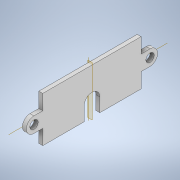
# Autodesk Inventor part: pokrywa_baza
Saved by Autodesk Inventor 2021 (Build 250183000, 183)
## iProperties
Created: 2025-11-29
Part Number: pokrywa_baza
Material: Generic
Document SubType Name: Modeling
Designer: huber
Density: 1 g/cm^3
Appearance: Default
Author: huber
Autodesk Inventor part; units mm, degrees
ref_plane "YZ Plane" through (0, 0, 0) normal (1, 0, 0) x (0, 1, 0)
ref_plane "XZ Plane" through (0, 0, 0) normal (0, 1, 0) x (-1, 0, 0)
sketch "Sketch1" plane through (0, 0, 0) normal (1, 0, 0) x (0, 1, 0)
  line L0 (11.5, 25) -> (-11.5, 25)
  line L1 (-11.5, 25) -> (-11.5, -25)
  line L2 (-11.5, -25) -> (11.5, -25)
  line L3 (11.5, -25) -> (11.5, 25)
  line L4 (11.5, 25) -> (-11.5, -25) construction
  line L5 (-11.5, 25) -> (11.5, -25) construction
  circle A0 centre (0, -29.5) radius 3.875
  line L6 (3.875, -29.5) -> (3.875, -25)
  line L7 (-3.875, -29.5) -> (-3.875, -25)
  line L8 (0, -45.05) -> (0, 36.675) projected
  circle A1 centre (0, -29.5) radius 2.1
  line L9 (-16.1, 0) -> (16.1, 0) projected
  circle A2 centre (-4.5, 0) radius 4
  line L10 (-4.5, 4) -> (-11.5, 4)
  line L11 (-4.5, -4) -> (-11.5, -4)
  point P0 (0, 0)
  point P1 (-11.5, 1.75)
  point P2 (-11.5, -4.25)
  point P3 (4, 25)
  point P4 (-4, 25)
  dimension "d0" = 50
  dimension "d1" = 23
  dimension "d4" = 7.75
  dimension "d5" = 4.5
  dimension "d6" = 4.2
  dimension "d11" = 8
  dimension "d12" = 7
  constraints: 20 end point, 10 point on line, 5 perpendicular, 4 point on circle, 4 tangent, 3 centre point, 2 midpoint, 2 parallel, 1 coincident, 1 horizontal
  measures "d0" distance of L0.end L1.end
  measures "d1" distance of L1.end L2.end
  measures "d4" diameter of A0
  measures "d5" distance from line of L2 A0.centre
  measures "d6" diameter of A1
  measures "d11" diameter of A2
  measures "d12" distance from line of L1 A2.centre
extrude "Extrusion1" add sketch "Sketch1" along normal blind 2 contours L3 L9 L8 L0 | L8 L9 A2 L10 L1 L0 | L3 L2 L8 L9 | L8 L2 L1 L11 A2 L9 | L8 A0 L7 L2 | L2 L6 A0 L8 | L8 A1 A0 | A0 L8 A1
mirror "Mirror1" about plane through (0, 0, 0) normal (0, 0, 1) of "Extrusion1"
body "Solid1"
